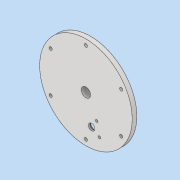
# Autodesk Inventor part: ThrustBearingMount
Saved by Autodesk Inventor 2017 (Build 210142000, 142)
## iProperties
Created: 2016-11-30
Part Number: ThrustBearingMount
Material: ABS Plastic
Document SubType Name: Modeling
Designer: techn
Density: 1.06 g/cm^3
Appearance: Smooth - White
Author: techn
Autodesk Inventor part; units mm, degrees
ref_plane "YZ Plane" through (0, 0, 0) normal (1, 0, 0) x (0, 1, 0)
ref_plane "XZ Plane" through (0, 0, 0) normal (0, 1, 0) x (-1, 0, 0)
ref_plane "XY Plane" through (0, 0, 0) normal (0, 0, 1) x (1, 0, 0)
sketch "Sketch5" plane through (0, 0, 0) normal (0, 0, 1) x (1, 0, 0)
  circle A0 centre (0, 0) radius 47.625
  dimension "d15" = 95.25
  constraints: 1 centre point, 1 coincident
  measures "d15" diameter of A0
extrude "Extrusion3" add sketch "Sketch5" along normal blind 4.7625
sketch "Sketch6" plane through (0, 0, 4.7625) normal (0, 0, 1) x (1, 0, 0)
  line L0 (0, 0) -> (0, 41.91)
  circle A0 centre (0, 41.91) radius 1.5875
  circle A1 centre (-36.2951, 20.955) radius 1.5875
  circle A2 centre (-36.2951, -20.955) radius 1.5875
  circle A3 centre (0, -41.91) radius 1.5875
  circle A4 centre (36.2951, -20.955) radius 1.5875
  circle A5 centre (36.2951, 20.955) radius 1.5875
  dimension "d18" = 41.91
  dimension "d19" = 3.175
  dimension "d22" = 360
  constraints: 6 centre point, 2 end point, 1 coincident, 1 vertical, 13 other
  measures "d18" distance of L0.start L0.end
  measures "d19" diameter of A0
extrude "Extrusion4" cut sketch "Sketch6" against normal blind 4.7625
sketch "Sketch7" plane through (0, 0, 0) normal (0, 0, -1) x (-1, 0, 0)
  circle A0 centre (0, 0) radius 11.303
  circle A1 centre (0, 0) radius 14.2875
  dimension "d26" = 22.606
  dimension "d27" = 28.575
  constraints: 2 centre point, 2 coincident
  measures "d26" diameter of A0
  measures "d27" diameter of A1
extrude "Extrusion5" add sketch "Sketch7" along normal blind 3.6068
sketch "Sketch9" plane through (0, 0, 0) normal (0, 0, -1) x (-1, 0, 0)
  circle A0 centre (0, 0) radius 4.7625
  dimension "d30" = 9.525
  constraints: 1 centre point, 1 coincident
  measures "d30" diameter of A0
extrude "Extrusion6" cut sketch "Sketch9" against normal through all
sketch "Sketch10" plane through (0, 0, 0) normal (0, 0, -1) x (-1, 0, 0)
  circle A0 centre (0, 0) radius 4.7625
  circle A1 centre (0, 0) radius 6.096
  dimension "d33" = 9.525
  dimension "d34" = 12.192
  constraints: 2 centre point, 2 coincident
  measures "d33" diameter of A0
  measures "d34" diameter of A1
extrude "Extrusion7" add sketch "Sketch10" along normal blind 3.6068
sketch "Sketch14" plane through (0, 0, 4.7625) normal (0, 0, 1) x (1, 0, 0)
  circle A0 centre (0, 0) radius 4.7625 projected
  line L0 (0, 0) -> (5.9411, -27.9506)
  line L1 (0, 0) -> (28.575, 0) construction
  line L2 (5.9411, -27.9506) -> (11.1288, -19.9622)
  line L3 (5.9411, -27.9506) -> (15.4661, -27.9506) construction
  circle A1 centre (11.1288, -19.9622) radius 1.27
  circle A2 centre (-2.0473, -22.7629) radius 1.27
  circle A3 centre (0.7534, -35.9389) radius 1.27
  circle A4 centre (13.9294, -33.1383) radius 1.27
  circle A5 centre (5.9411, -27.9506) radius 3.302
  dimension "d60" = 28.575
  dimension "d61" = 78
  dimension "d62" = 9.525
  dimension "d64" = 2.54
  dimension "d67" = 360
  dimension "d69" = 6.604
  dimension "d75" = 45
  constraints: 8 end point, 5 centre point, 2 coincident, 2 equal length, 2 horizontal, 9 other
  measures "d60" distance of L0.start L0.end
  measures "d61" angle of L0 L1
  measures "d62" distance of L0.end L2.end
  measures "d64" diameter of A1
  measures "d69" diameter of A5
  measures "d75" angle of L2 L0
extrude "Extrusion14" cut sketch "Sketch14" against normal blind 25.4 contours A5 L2 L0 | L0 L2 A5 | A1 | A4
sketch "Sketch16" plane through (0, 0, 0) normal (0, 0, -1) x (-1, 0, 0)
  circle A0 centre (-5.9411, -27.9506) radius 3.302 projected
  circle A1 centre (-5.9411, -27.9506) radius 6.35
  point P0 (0, 0)
  dimension "d78" = 12.7
  constraints: 1 centre point, 1 coincident
  measures "d78" diameter of A1
extrude "Extrusion15" cut sketch "Sketch16" against normal blind 3.175
body "Solid2"
